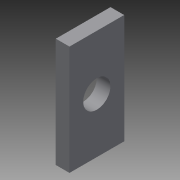
# Autodesk Inventor part: CatapultArmSquare-Thickener
Saved by Autodesk Inventor 2013 (Build 170138000, 138)
## iProperties
Created: 2014-01-20
Part Number: CatapultArmSquare-Thickener
Material: Generic
Document SubType Name: Modeling
Designer: RobertB
Density: 1 g/cm^3
Author: RobertB
Autodesk Inventor part; units mm, degrees
ref_plane "YZ Plane" through (0, 0, 0) normal (1, 0, 0) x (0, 1, 0)
ref_plane "XZ Plane" through (0, 0, 0) normal (0, 1, 0) x (-1, 0, 0)
ref_plane "XY Plane" through (0, 0, 0) normal (0, 0, 1) x (1, 0, 0)
sketch "Sketch1" plane through (0, 0, 0) normal (1, 0, 0) x (0, 1, 0)
  line L0 (0, 0) -> (114.3, 0)
  line L1 (114.3, 0) -> (114.3, 25.4)
  line L2 (114.3, 25.4) -> (0, 25.4)
  line L3 (0, 25.4) -> (0, 0)
  line L4 (114.3, 12.7) -> (88.9, 12.7)
  line L5 (88.9, 12.7) -> (25.4, 12.7)
  circle A0 centre (25.4, 12.7) radius 6.35
  circle A1 centre (88.9, 12.7) radius 6.35
  dimension "d0" = 114.3
  dimension "d1" = 25.4
  dimension "d4" = 25.4
  dimension "d5" = 63.5
  dimension "d6" = 12.7
  dimension "d7" = 12.7
  constraints: 12 end point, 2 centre point, 2 coincident, 2 parallel, 2 perpendicular, 1 collinear, 1 horizontal, 1 midpoint
  measures "d0" distance of L2.end L1.end
  measures "d1" distance of L1.end L0.end
  measures "d4" distance of L4.start L4.end
  measures "d5" distance of L4.end L5.end
  measures "d6" diameter of A0
  measures "d7" diameter of A1
extrude "Extrusion2" add sketch "Sketch1" along normal blind 6.35
body "Solid2"
